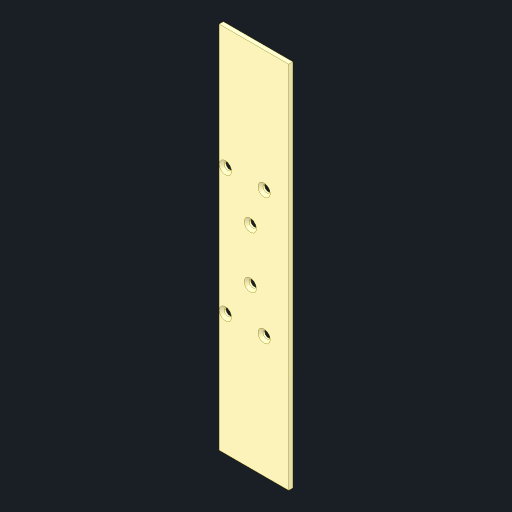
# Autodesk Inventor part: back
Saved by Autodesk Inventor 2023 (Build 270158000, 158)
## iProperties
Created: 2024-04-30
Part Number: back
Material: Nylon 6/6
Document SubType Name: Modeling
Designer: szymo
Density: 1.13 g/cm^3
Appearance: Nylon 6
Mass: 9.46005 g
Surface Area: 144.422 cm^2
Volume: 8.37172 cm^3
Author: szymo
Autodesk Inventor part; units mm, degrees
ref_plane "YZ Plane" through (0, 0, 0) normal (1, 0, 0) x (0, 1, 0)
ref_plane "XZ Plane" through (0, 0, 0) normal (0, 1, 0) x (-1, 0, 0)
ref_plane "XY Plane" through (0, 0, 0) normal (0, 0, 1) x (1, 0, 0)
ref_plane "Work Plane1" through (0, 0, 0) normal (0, 0, 1) x (1, 0, 0)
sketch "Sketch1" plane through (0, 0, 0) normal (0, 0, 1) x (1, 0, 0)
  line L0 (0, 0) -> (0, 68) projected
  line L1 (0, 68) -> (-3.5, 68) projected
  line L2 (-3.5, 0) -> (-3.5, 68) projected
  line L3 (0, 0) -> (-3.5, 0) projected
  line L4 (-3.5, 7) -> (-3.5, 0) projected
  line L5 (-3.5, 7) -> (-33.5, 7) projected
  line L6 (-33.5, 7) -> (-33.5, 0) projected
  line L7 (-6.5, 0) -> (-33.5, 0) projected
  line L8 (-3.5, 0) -> (-6.5, 0) projected
  line L9 (-33.5, 19) -> (-33.5, 24) projected
  line L10 (-33.5, 19) -> (-3.5, 19) projected
  line L11 (-3.5, 19) -> (-3.5, 24) projected
  line L12 (-3.5, 24) -> (-33.5, 24) projected
  line L13 (-33.5, 49) -> (-33.5, 44) projected
  line L14 (-3.5, 44) -> (-33.5, 44) projected
  line L15 (-3.5, 49) -> (-3.5, 44) projected
  line L16 (-33.5, 49) -> (-3.5, 49) projected
  line L17 (-3.5, 61) -> (-3.5, 68) projected
  line L18 (-3.5, 68) -> (-6.5, 68) projected
  line L19 (-6.5, 68) -> (-33.5, 68) projected
  line L20 (-33.5, 61) -> (-33.5, 68) projected
  line L21 (-3.5, 61) -> (-33.5, 61) projected
  line L22 (-34.5, 123) -> (10.5, 123) projected
  line L23 (10.5, -55) -> (-34.5, -55) projected
  line L24 (-33.5, 123) -> (-33.5, -55.3182)
  circle A0 centre (-30.5, 64.5) radius 2.3 projected
  circle A1 centre (-11.8324, 64.5) radius 2.3 projected
  circle A2 centre (-18.5, 21.5) radius 2.3 projected
  circle A3 centre (-18.5, 46.5) radius 2.3 projected
  line L25 (0, -55) -> (0, 123)
  point P0 (-33.5, -55)
  dimension "d10" = 0
  dimension "d41" = 0
  constraints: 4 end point, 3 point on line, 2 perpendicular
  measures "d10" distance between parallel lines of L0 L25
  measures "d41" distance between parallel lines of L24 L9
extrude "Extrusion1" add sketch "Sketch1" along normal blind 2 contours L3 L2 L1 L0 | L25 L23 L24 L7 L8 L3 | L1 L18 L19 L24 L22 L25 | L8 L7 L6 L5 L2 | L2 L21 L20 L19 L18 | L5 L24 L10 L2 | L2 L16 L24 L21 | L10 L9 L12 L2 | L2 L14 L13 L16 | L12 L24 L14 L2 | A0 | A1 | A2 | A3
sketch "Sketch2" plane through (0, 0, 2) normal (0, 0, 1) x (1, 0, 0)
  circle A0 centre (-30.5, 3.5) radius 2.3 projected
  circle A1 centre (-11.8324, 3.5) radius 2.3 projected
  line L0 (-3.5, 7) -> (-3.5, 0) projected
  line L1 (-3.5, 7) -> (-33.5, 7) projected
  line L2 (-33.5, 7) -> (-33.5, 0) projected
  line L3 (-6.5, 0) -> (-33.5, 0) projected
  line L4 (-3.5, 0) -> (-6.5, 0) projected
  circle A2 centre (-18.5, 46.5) radius 2.3 projected
  line L5 (-33.5, 49) -> (-33.5, 44) projected
  line L6 (-3.5, 44) -> (-33.5, 44) projected
  line L7 (-3.5, 49) -> (-3.5, 44) projected
  line L8 (-33.5, 49) -> (-3.5, 49) projected
  circle A3 centre (-18.5, 21.5) radius 2.3 projected
  line L9 (-33.5, 19) -> (-33.5, 24) projected
  line L10 (-33.5, 19) -> (-3.5, 19) projected
  line L11 (-3.5, 19) -> (-3.5, 24) projected
  line L12 (-3.5, 24) -> (-33.5, 24) projected
  circle A4 centre (-30.5, 64.5) radius 2.3 projected
  circle A5 centre (-11.8324, 64.5) radius 2.3 projected
  line L13 (-3.5, 61) -> (-3.5, 68) projected
  line L14 (-3.5, 68) -> (-6.5, 68) projected
  line L15 (-6.5, 68) -> (-33.5, 68) projected
  line L16 (-33.5, 61) -> (-33.5, 68) projected
  line L17 (-3.5, 61) -> (-33.5, 61) projected
  point P0 (0, 0)
  constraints: 6 coincident
hole "Hole1" at (-30.5, 3.5, 2) at (-11.8324, 3.5, 2) at (-18.5, 21.5, 2) at (-18.5, 46.5, 2) at (-30.5, 64.5, 2) at (-11.8324, 64.5, 2) direction (0, 0, -1) diameter 3.6 end through all countersink diameter 6 countersink angle 90 clearance for "Countersunk Flat Head Screw ISO 2009/7046" size "M3" standard "ISO"
sketch "Sketch3" plane through (0, 0, 0) normal (0, 0, -1) x (-1, 0, 0)
  circle A0 centre (30.5, 3.5) radius 2.3 projected
  circle A1 centre (11.8324, 3.5) radius 2.3 projected
  line L0 (3.5, 7) -> (3.5, 0) projected
  line L1 (3.5, 7) -> (33.5, 7) projected
  line L2 (33.5, 7) -> (33.5, 0) projected
  line L3 (6.5, 0) -> (33.5, 0) projected
  line L4 (3.5, 0) -> (6.5, 0) projected
  circle A2 centre (18.5, 21.5) radius 2.3 projected
  line L5 (33.5, 19) -> (33.5, 24) projected
  line L6 (33.5, 19) -> (3.5, 19) projected
  line L7 (3.5, 19) -> (3.5, 24) projected
  line L8 (3.5, 24) -> (33.5, 24) projected
  circle A3 centre (18.5, 46.5) radius 2.3 projected
  line L9 (33.5, 49) -> (33.5, 44) projected
  line L10 (3.5, 44) -> (33.5, 44) projected
  line L11 (3.5, 49) -> (3.5, 44) projected
  line L12 (33.5, 49) -> (3.5, 49) projected
  circle A4 centre (30.5, 64.5) radius 2.3 projected
  circle A5 centre (11.8324, 64.5) radius 2.3 projected
  line L13 (3.5, 61) -> (3.5, 68) projected
  line L14 (3.5, 68) -> (6.5, 68) projected
  line L15 (6.5, 68) -> (33.5, 68) projected
  line L16 (33.5, 61) -> (33.5, 68) projected
  line L17 (3.5, 61) -> (33.5, 61) projected
  line L18 (34.5, 123) -> (34.5, -55) projected
  line L19 (34.5, 68) -> (0, 68)
  line L20 (0, 68) -> (0, 0)
  line L21 (0, 0) -> (34.5, 0)
  line L22 (34.5, 0) -> (34.5, 68)
  line L23 (32.5, 68) -> (2, 68)
  line L24 (2, 68) -> (2, 121)
  line L25 (2, 121) -> (32.5, 121)
  line L26 (32.5, 121) -> (32.5, 68)
  line L27 (32.5, 0) -> (2, 0)
  line L28 (2, 0) -> (2, -53)
  line L29 (2, -53) -> (32.5, -53)
  line L30 (32.5, -53) -> (32.5, 0)
  line L31 (0, 123) -> (33.5, 123) projected
  line L32 (0, -55) -> (0, 123) projected
  line L33 (33.5, -55) -> (0, -55) projected
  line L34 (2, 68) -> (32.5, 121) construction
  line L35 (32.5, 68) -> (2, 121) construction
  line L36 (32.5, 0) -> (2, -53) construction
  line L37 (32.5, -53) -> (2, 0) construction
  line L38 (3.1538, 121) -> (32.5, 70.0049)
  line L39 (2, 118.9951) -> (31.3462, 68)
  line L40 (3.1538, 68) -> (32.5, 118.9951)
  line L41 (31.3462, 121) -> (2, 70.0049)
  line L42 (3.1538, 0) -> (32.5, -50.9951)
  line L43 (31.3462, -53) -> (2, -2.0049)
  line L44 (2, -50.9951) -> (31.3462, 0)
  line L45 (32.5, -2.0049) -> (3.1538, -53)
  line L46 (32.5, 61) -> (2, 61)
  line L47 (2, 61) -> (2, 49)
  line L48 (2, 49) -> (32.5, 49)
  line L49 (32.5, 49) -> (32.5, 61)
  line L50 (32.5, 44) -> (2, 44)
  line L51 (2, 44) -> (2, 24)
  line L52 (2, 24) -> (32.5, 24)
  line L53 (32.5, 24) -> (32.5, 44)
  line L54 (32.5, 19) -> (2, 19)
  line L55 (2, 19) -> (2, 7)
  line L56 (2, 7) -> (32.5, 7)
  line L57 (32.5, 7) -> (32.5, 19)
  line L58 (32.5, 61) -> (2, 49) construction
  line L59 (32.5, 49) -> (2, 61) construction
  line L60 (2, 44) -> (32.5, 24) construction
  line L61 (32.5, 44) -> (2, 24) construction
  line L62 (2, 19) -> (32.5, 7) construction
  line L63 (32.5, 19) -> (2, 7) construction
  line L64 (2, 50.0746) -> (29.7687, 61)
  line L65 (32.5, 59.9254) -> (4.7313, 49)
  line L66 (32.5, 50.0746) -> (4.7313, 61)
  line L67 (2, 59.9254) -> (29.7687, 49)
  line L68 (30.6764, 44) -> (2, 25.1958)
  line L69 (32.5, 42.8042) -> (3.8236, 24)
  line L70 (2, 42.8042) -> (30.6764, 24)
  line L71 (32.5, 25.1958) -> (3.8236, 44)
  line L72 (32.5, 17.9254) -> (4.7313, 7)
  line L73 (2, 8.0746) -> (29.7687, 19)
  line L74 (4.7313, 19) -> (32.5, 8.0746)
  line L75 (29.7687, 7) -> (2, 17.9254)
  point P0 (17.25, -24.4951)
  point P1 (31.3462, 0)
  point P2 (18.4038, -26.5)
  point P3 (17.25, -28.5049)
  point P4 (16.0962, -26.5)
  point P5 (17.25, 92.4951)
  point P6 (16.0962, 94.5)
  point P7 (18.4038, 94.5)
  point P8 (17.25, 96.5049)
  point P9 (19.9813, 13)
  point P10 (17.25, 11.9254)
  point P11 (4.7313, 7)
  point P12 (14.5187, 13)
  point P13 (17.25, 14.0746)
  point P14 (17.25, 32.8042)
  point P15 (3.8236, 24)
  point P16 (19.0736, 34)
  point P17 (15.4264, 34)
  point P18 (3.8236, 44)
  point P19 (17.25, 35.1958)
  point P20 (14.5187, 55)
  point P21 (4.7313, 49)
  point P22 (17.25, 56.0746)
  point P23 (19.9813, 55)
  point P24 (17.25, 53.9254)
  dimension "d11" = 2
  dimension "d12" = 2
  dimension "d13" = 2
  dimension "d14" = 2
  dimension "d15" = 2
  dimension "d16" = 2
  dimension "d17" = 1
  dimension "d18" = 1
  dimension "d19" = 1
  dimension "d20" = 1
  dimension "d21" = 1
  dimension "d22" = 1
  dimension "d23" = 1
  dimension "d24" = 1
  dimension "d27" = 2
  dimension "d28" = 2
  dimension "d29" = 1
  dimension "d30" = 1
  dimension "d31" = 1
  dimension "d32" = 1
  dimension "d33" = 1
  dimension "d34" = 1
  dimension "d35" = 1
  dimension "d36" = 1
  dimension "d37" = 1
  dimension "d38" = 1
  dimension "d39" = 1
  dimension "d40" = 1
  constraints: 108 end point, 54 point on line, 33 parallel, 6 horizontal, 6 perpendicular, 1 collinear
  measures "d11" distance between parallel lines of L18 L26
  measures "d12" distance between parallel lines of L31 L25
  measures "d13" distance between parallel lines of L24 L32
  measures "d14" distance between parallel lines of L32 L28
  measures "d15" distance between parallel lines of L18 L30
  measures "d16" distance between parallel lines of L33 L29
  measures "d17" distance between parallel lines of L36 L45
  measures "d18" distance between parallel lines of L36 L44
  measures "d19" distance between parallel lines of L37 L42
  measures "d20" distance between parallel lines of L37 L43
  measures "d21" distance between parallel lines of L38 L35
  measures "d22" distance between parallel lines of L35 L39
  measures "d23" distance between parallel lines of L34 L40
  measures "d24" distance between parallel lines of L34 L41
  measures "d27" distance between parallel lines of L47 L20
  measures "d28" distance between parallel lines of L22 L49
  measures "d29" distance between parallel lines of L58 L65
  measures "d30" distance between parallel lines of L58 L64
  measures "d31" distance between parallel lines of L59 L66
  measures "d32" distance between parallel lines of L59 L67
  measures "d33" distance between parallel lines of L61 L69
  measures "d34" distance between parallel lines of L61 L68
  measures "d35" distance between parallel lines of L60 L71
  measures "d36" distance between parallel lines of L60 L70
  measures "d37" distance between parallel lines of L63 L73
  measures "d38" distance between parallel lines of L63 L72
  measures "d39" distance between parallel lines of L62 L74
  measures "d40" distance between parallel lines of L62 L75
extrude "Extrusion2" cut sketch "Sketch3" against normal blind 1 contours L4 L3 L44 L42 L21 | L72 L75 L1 | L55 L75 L73 | L72 L57 L74 | L43 L44 L28 | L45 L30 L42 | L74 L6 L73 | L43 L29 L45 | L40 L39 L15 L14 L19 | L24 L39 L41 | L69 L70 L8 | L51 L70 L68 | L40 L26 L38 | L38 L25 L41 | L71 L69 L53 | L17 L64 L66 | L71 L10 L68 | L49 L66 L65 | L67 L64 L47 | L67 L12 L65
body "Solid1"
